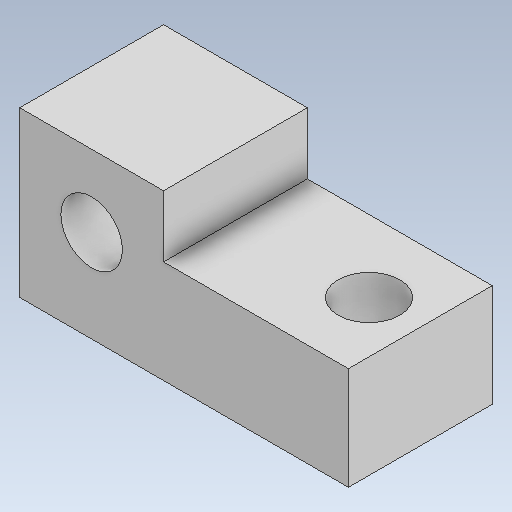
# Autodesk Inventor part: angle_01
Saved by Autodesk Inventor 2020 (Build 240168000, 168)
## iProperties
Created: 2024-02-24
Part Number: angle_01
Material: Типовые
Document SubType Name: Modeling
Designer: 4s
Density: 1 g/cm^3
Appearance: По умолчанию
Author: 4s
Autodesk Inventor part; units mm, degrees
ref_plane "YZ Plane" through (0, 0, 0) normal (1, 0, 0) x (0, 1, 0)
ref_plane "XZ Plane" through (0, 0, 0) normal (0, 1, 0) x (-1, 0, 0)
ref_plane "XY Plane" through (0, 0, 0) normal (0, 0, 1) x (1, 0, 0)
sketch "Эскиз1" plane through (0, 0, 0) normal (0, 1, 0) x (-1, 0, 0)
  line L0 (0, 0) -> (-16, 0)
  line L1 (-16, 0) -> (-16, -7)
  line L2 (-16, -7) -> (0, -7)
  line L3 (0, -7) -> (0, 0)
  circle A0 centre (-13.5, -3.5) radius 1.5
  dimension "d0" = 16
  dimension "d1" = 7
  dimension "d2" = 3
  dimension "d3" = 2.5
  dimension "d4" = 3.5
  constraints: 8 end point, 2 parallel, 1 centre point, 1 horizontal, 1 perpendicular
  measures "d0" distance of L1.end L2.end
  measures "d1" distance of L0.end L1.end
  measures "d2" diameter of A0
  measures "d3" distance from line of L1 A0.centre
  measures "d4" distance from line of L0 A0.centre
extrude "Выдавливание1" add sketch "Эскиз1" along normal blind 5
sketch "Эскиз2" plane through (0, 0, 0) normal (0, 1, 0) x (-1, 0, 0)
  line L0 (-16, 0) -> (-16, -7) construction
  line L1 (-16, -7) -> (0, -7) construction
  line L2 (0, -7) -> (0, 0) projected
  line L3 (0, 0) -> (-16, 0) construction
  circle A0 centre (-13.5, -3.5) radius 1.5 construction
  line L4 (0, 0) -> (-7, 0)
  line L5 (-7, 0) -> (-7, -7)
  line L6 (-7, -7) -> (0, -7)
  line L7 (0, -7) -> (0, 0)
  point P0 (0, -7)
  dimension "d7" = 7
  dimension "d8" = 7
  constraints: 8 end point, 2 parallel, 1 horizontal, 1 perpendicular
  measures "d7" distance of L6.end L5.end
  measures "d8" distance of L5.end L4.end
extrude "Выдавливание2" add sketch "Эскиз2" along normal blind 8
sketch "Эскиз3" plane through (0, 0, 0) normal (0, 0, 1) x (1, 0, 0)
  line L0 (0, 0) -> (16, 0) construction
  line L1 (16, 0) -> (16, 5) construction
  line L2 (7, 5) -> (16, 5) construction
  line L3 (7, 5) -> (7, 8) construction
  line L4 (0, 8) -> (7, 8) construction
  line L5 (0, 0) -> (0, 8) construction
  circle A0 centre (3.5, 4.5) radius 1.5
  dimension "d11" = 3
  dimension "d12" = 3.5
  dimension "d13" = 3.5
  constraints: 1 centre point
  measures "d11" diameter of A0
  measures "d12" distance from line of L4 A0.centre
  measures "d13" distance from line of L5 A0.centre
extrude "Выдавливание3" cut sketch "Эскиз3" against normal blind 7
